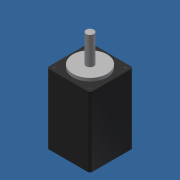
# Autodesk Inventor part: Nema11
Saved by Autodesk Inventor 2014 SP2 (Build 180246200, 246)
## iProperties
Created: 2014-12-14
Part Number: Nema11
Material: Stahl
Document SubType Name: Modeling
Designer: 4ndreas
Density: 7.85 g/cm^3
Appearance: Stahl
Mass: 284.49 g
Surface Area: 70.7835 cm^2
Volume: 36.2408 cm^3
Author: 4ndreas
Autodesk Inventor part; units mm, degrees
ref_plane "YZ Plane" through (0, 0, 0) normal (1, 0, 0) x (0, 1, 0)
ref_plane "XZ Plane" through (0, 0, 0) normal (0, 1, 0) x (-1, 0, 0)
ref_plane "XY Plane" through (0, 0, 0) normal (0, 0, 1) x (1, 0, 0)
sketch "Skizze1" plane through (0, 0, 0) normal (0, 0, 1) x (1, 0, 0)
  line L0 (-14, 14) -> (14, 14)
  line L1 (14, 14) -> (14, -14)
  line L2 (14, -14) -> (-14, -14)
  line L3 (-14, -14) -> (-14, 14)
  circle A0 centre (0, 0) radius 11
  circle A1 centre (0, 0) radius 2.5
  line L4 (-14, 0) -> (14, 0) construction
  line L5 (0, 14) -> (0, -14) construction
  line L6 (-11.4905, 11.4905) -> (11.4905, 11.4905) construction
  line L7 (11.4905, 11.4905) -> (11.4905, -11.4905) construction
  line L8 (11.4905, -11.4905) -> (-11.4905, -11.4905) construction
  line L9 (-11.4905, -11.4905) -> (-11.4905, 11.4905) construction
  circle A2 centre (0, 0) radius 16.25 construction
  point P0 (0, -11.4905)
  point P1 (11.4905, 0)
  dimension "d4" = 32.5
  dimension "d0" = 5
  dimension "d1" = 22
  dimension "d2" = 28
  constraints: 20 end point, 8 midpoint, 5 coincident, 4 parallel, 4 perpendicular, 2 centre point, 2 horizontal, 2 point on line, 3 other
  measures "d0" diameter of A1
  measures "d1" diameter of A0
  measures "d2" distance between parallel lines of L1 L3
extrude "Extrusion1" add sketch "Skizze1" along normal blind 2 contours A0 | A1
extrude "Extrusion2" add sketch "Skizze1" along normal blind 20 contours A1
extrude "Extrusion3" add sketch "Skizze1" against normal blind 45 contours L0 L1 L2 L3 | A0 | A1
hole "Bohrung1" at (-11.4905, 11.4905, 0) at (11.4905, 11.4905, 0) at (11.4905, -11.4905, 0) at (-11.4905, -11.4905, 0) direction (0, 0, -1) diameter 1.567 depth 8 tip angle 118 thread size "M2x0.4" class "6H" standard "ANSI Metric M Profile"
chamfer "Fase1" distance 1 angle 45 4 edges at (14, -14, -22.5) (-14, -14, -22.5) (14, 14, -22.5) (-14, 14, -22.5)
